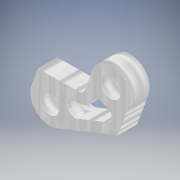
# Autodesk Inventor part: アーム先端返し抑え1
Saved by Autodesk Inventor 2020 (Build 240168000, 168)
## iProperties
Created: 2019-08-05
Part Number: アーム先端返し抑え1
Material: アルミニウム 7075
Document SubType Name: Modeling
Designer: 雪村
Density: 2.81 g/cm^3
Appearance: サテン - ブラシ仕上げ 重厚
Mass: 0.629939 g
Surface Area: 3.95681 cm^2
Volume: 0.224178 cm^3
Description: アルミ7000 3t
Author: 雪村
Autodesk Inventor part; units mm, degrees
ref_plane "YZ Plane" through (0, 0, 0) normal (1, 0, 0) x (0, 1, 0)
ref_plane "XZ Plane" through (0, 0, 0) normal (0, 1, 0) x (-1, 0, 0)
ref_plane "XY Plane" through (0, 0, 0) normal (0, 0, 1) x (1, 0, 0)
sketch "スケッチ1" plane through (0, 0, 0) normal (0, 0, 1) x (1, 0, 0)
  circle A0 centre (-170.8124, -0.9741) radius 1.5
  circle A1 centre (-161.3061, 5.8993) radius 1.5
  circle A2 centre (-161.3061, 5.8993) radius 3
  circle A3 centre (-170.8124, -0.9741) radius 3
  line L0 (-160.252, 0.0251) -> (-151.4456, 24.2153)
  arc A4 (-162.6881, 3.2366) -> (-161.9719, 2.9741) centre (-161.3061, 5.8993) ccw
  arc A5 (-161.2542, 1.657) -> (-161.9719, 2.9741) centre (-162.1939, 1.9991) ccw
  line L1 (-161.2542, 1.657) -> (-161.2792, 1.5882)
  arc A6 (-161.847, 1.002) -> (-161.2792, 1.5882) centre (-162.2189, 1.9303) ccw
  line L2 (-161.847, 1.002) -> (-166.5706, -0.8906)
  arc A7 (-167.91, -0.2153) -> (-166.5706, -0.8906) centre (-166.9425, 0.0377) ccw
  arc A8 (-167.91, -0.2153) -> (-167.9841, 0.0261) centre (-170.8124, -0.9741) ccw
  arc A9 (-167.0482, 1.3595) -> (-167.9841, 0.0261) centre (-167.0413, 0.3595) ccw
  line L3 (-167.0482, 1.3595) -> (-166.2863, 1.3648)
  arc A10 (-166.2863, 1.3648) -> (-164.0502, 2.7821) centre (-166.3036, 3.8647) ccw
  arc A11 (-162.6881, 3.2366) -> (-164.0502, 2.7821) centre (-163.1488, 2.3491) ccw
  arc A12 (-157.2727, 21.3635) -> (-159.6219, 24.7187) centre (-159.6219, 22.2187) ccw
  line L4 (-159.6219, 24.7187) -> (-161.4168, 24.7187)
  arc A13 (-162.3541, 26.0674) -> (-161.4168, 24.7187) centre (-161.4168, 25.7187) ccw
  line L5 (-162.3541, 26.0674) -> (-162.2502, 26.3466)
  arc A14 (-150.3521, 39.3594) -> (-162.2502, 26.3466) centre (-140.2247, 18.1536) ccw
  arc A15 (-149.1659, 37.8016) -> (-150.3521, 39.3594) centre (-149.9212, 38.457) ccw
  arc A16 (-149.1659, 37.8016) -> (-153.03, 24.598) centre (-136.7039, 26.9873) ccw
  arc A17 (-153.0798, 24.1111) -> (-153.03, 24.598) centre (-154.0195, 24.4532) ccw
  line L6 (-153.0798, 24.1111) -> (-158.539, 9.1154)
  arc A18 (-159.9355, 8.5679) -> (-158.539, 9.1154) centre (-159.4786, 9.4575) ccw
  arc A19 (-159.9355, 8.5679) -> (-160.7114, 8.8398) centre (-161.3061, 5.8993) ccw
  arc A20 (-161.5067, 9.9339) -> (-160.7114, 8.8398) centre (-160.5132, 9.82) ccw
  arc A21 (-161.5067, 9.9339) -> (-162.0534, 11.7992) centre (-163.9904, 10.2187) ccw
  arc A22 (-161.4656, 13.4137) -> (-162.0534, 11.7992) centre (-161.2785, 12.4313) ccw
  arc A23 (-161.4656, 13.4137) -> (-159.5841, 15.0143) centre (-161.9333, 15.8696) ccw
  line L7 (-159.5841, 15.0143) -> (-159.457, 15.3635)
  arc A24 (-159.457, 15.3635) -> (-159.8691, 17.7992) centre (-161.8061, 16.2187) ccw
  arc A25 (-159.2813, 19.4137) -> (-159.8691, 17.7992) centre (-159.0943, 18.4313) ccw
  arc A26 (-159.2813, 19.4137) -> (-157.3998, 21.0143) centre (-159.749, 21.8696) ccw
  line L8 (-157.3998, 21.0143) -> (-157.2727, 21.3635)
  circle A27 centre (-170.8124, -0.9741) radius 1.5
  circle A28 centre (-161.3061, 5.8993) radius 1.5
  arc A29 (-173.6242, 0.0718) -> (-169.6967, -3.7589) centre (-170.8124, -0.9741) ccw
  line L9 (-169.6967, -3.7589) -> (-160.252, 0.0251)
  line L10 (-160.252, 0.0251) -> (-151.4456, 24.2153)
  arc A30 (-141.6605, 41.1447) -> (-151.4456, 24.2153) centre (-136.7039, 26.9873) ccw
  arc A31 (-141.6605, 41.1447) -> (-142.0645, 43.0859) centre (-141.9909, 42.0886) ccw
  arc A32 (-142.0645, 43.0859) -> (-163.6561, 26.8696) centre (-140.2247, 18.1536) ccw
  line L11 (-163.6561, 26.8696) -> (-164.3351, 25.0441)
  line L12 (-164.3351, 25.0441) -> (-163.1936, 23.2187)
  line L13 (-163.1936, 23.2187) -> (-159.6219, 23.2187)
  arc A33 (-158.6822, 21.8766) -> (-159.6219, 23.2187) centre (-159.6219, 22.2187) ccw
  line L14 (-158.6822, 21.8766) -> (-158.8093, 21.5275)
  arc A34 (-159.749, 20.8696) -> (-158.8093, 21.5275) centre (-159.749, 21.8696) ccw
  line L15 (-159.749, 20.8696) -> (-164.0488, 20.8696)
  line L16 (-164.0488, 20.8696) -> (-166.567, 19.0441)
  line L17 (-166.567, 19.0441) -> (-165.3779, 17.2187)
  line L18 (-165.3779, 17.2187) -> (-161.8061, 17.2187)
  arc A35 (-160.8665, 15.8766) -> (-161.8061, 17.2187) centre (-161.8061, 16.2187) ccw
  line L19 (-160.8665, 15.8766) -> (-160.9936, 15.5275)
  arc A36 (-161.9333, 14.8696) -> (-160.9936, 15.5275) centre (-161.9333, 15.8696) ccw
  line L20 (-161.9333, 14.8696) -> (-166.2331, 14.8696)
  line L21 (-166.2331, 14.8696) -> (-168.7988, 13.0441)
  line L22 (-168.7988, 13.0441) -> (-167.5622, 11.2187)
  line L23 (-167.5622, 11.2187) -> (-163.9904, 11.2187)
  arc A37 (-163.0508, 9.8766) -> (-163.9904, 11.2187) centre (-163.9904, 10.2187) ccw
  line L24 (-163.0508, 9.8766) -> (-163.1779, 9.5275)
  arc A38 (-164.1175, 8.8696) -> (-163.1779, 9.5275) centre (-164.1175, 9.8696) ccw
  line L25 (-164.1175, 8.8696) -> (-168.4174, 8.8696)
  line L26 (-168.4174, 8.8696) -> (-171.0307, 7.0441)
  line L27 (-171.0307, 7.0441) -> (-169.7465, 5.1842)
  line L28 (-169.7465, 5.1842) -> (-166.1852, 5.2088)
  arc A39 (-165.2387, 3.8667) -> (-166.1852, 5.2088) centre (-166.1783, 4.2088) ccw
  line L29 (-165.2387, 3.8667) -> (-165.3639, 3.5226)
  arc A40 (-166.2967, 2.8648) -> (-165.3639, 3.5226) centre (-166.3036, 3.8647) ccw
  line L30 (-166.2967, 2.8648) -> (-172.6015, 2.8212)
  line L31 (-172.6015, 2.8212) -> (-173.6242, 0.0718)
  arc A41 (-165.2387, 3.8667) -> (-166.1852, 5.2088) centre (-166.1783, 4.2088) ccw
  line L32 (-164.1251, 6.9256) -> (-165.2387, 3.8667)
  point P0 (0, 0)
  point P1 (0, 0)
  point P2 (-158.4871, 4.8731)
  point P3 (-173.6242, 0.0718)
  point P4 (-169.6967, -3.7589)
  point P5 (-161.9719, 2.9741)
  point P6 (-167.91, -0.2153)
  point P7 (-167.9841, 0.0261)
  point P8 (-162.6881, 3.2366)
  constraints: 72 point on circle, 66 end point, 41 centre point, 7 horizontal, 2 coincident, 182 other
extrude "押し出し1" add sketch "スケッチ1" along normal blind 3 contours A2 | L0 L9 A3 A7 L2 A6 L1 A5 A2 | A2 A11 A10 L3 A9 A3 L31 L30 A40 L29 L32 | A3
